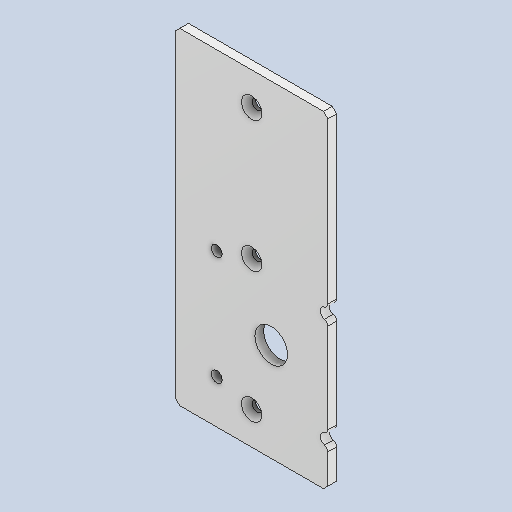
# Autodesk Inventor part: Espaçador módulo AC
Saved by Autodesk Inventor 2026 (Build 300175050, 175E)
## iProperties
Created: 2025-08-25
Part Number: Espaçador módulo AC
Material: Poliacetal
Document SubType Name: Modeling
Designer: Kedson Neves
Density: 1.41 g/cm^3
Appearance: Suave - Branco
Description: Espaçador módulo AC
Author: Kedson Neves
Autodesk Inventor part; units mm, degrees
ref_plane "YZ Plane" through (0, 0, 0) normal (1, 0, 0) x (0, 1, 0)
ref_plane "XZ Plane" through (0, 0, 0) normal (0, 1, 0) x (-1, 0, 0)
ref_plane "XY Plane" through (0, 0, 0) normal (0, 0, 1) x (1, 0, 0)
sketch "Esboço1" plane through (0, 0, 0) normal (0, 0, 1) x (1, 0, 0)
  line L0 (-35, -75) -> (35, -75)
  line L1 (35, -75) -> (35, 75)
  line L2 (35, 75) -> (-35, 75)
  line L3 (-35, 75) -> (-35, -75)
  line L4 (-35, -75) -> (35, 75) construction
  line L5 (35, -75) -> (-35, 75) construction
  point P0 (0, 0)
  dimension "d0" = 150
  dimension "d1" = 70
  constraints: 12 end point, 2 midpoint, 2 parallel, 1 horizontal, 1 perpendicular
  measures "d0" distance of L2.end L0.start
  measures "d1" distance of L1.end L2.end
extrude "Extrusão1" add sketch "Esboço1" along normal blind 4
sketch "Esboço2" plane through (0, 0, 4) normal (0, 0, 1) x (1, 0, 0)
  line L0 (35, 75) -> (-35, 75) projected
  line L1 (-35, -75) -> (35, -75) projected
  line L2 (-35, 75) -> (-35, -75) projected
  point P0 (0, 0)
  point P1 (0, 60)
  point P2 (0, -60)
  point P3 (0, 0)
  dimension "d4" = 15
  dimension "d5" = 15
  dimension "d6" = 35
  dimension "d7" = 35
  constraints: 1 coincident
  measures "d4" distance from line of L0 point (0, 60)
  measures "d5" distance from line of L1 point (0, -60)
  measures "d6" distance from line of L2 point (0, -60)
  measures "d7" distance from line of L2 point (0, 60)
hole "Furo1" at (0, 60, 4) at (0, -60, 4) at (0, 0, 4) direction (0, 0, -1) diameter 4.5 end through all countersink diameter 9.4 countersink angle 90 clearance for "Countersunk Flat Head Screw ISO 2009/7046" size "M4" standard "ISO"
chamfer "Chanfro1" distance 2 angle 45 4 edges at (35, -75, 2) (-35, -75, 2) (35, 75, 2) (-35, 75, 2)
sketch "Esboço3" plane through (0, 0, 4) normal (0, 0, 1) x (1, 0, 0)
  circle A0 centre (34, -55) radius 1.5706 projected
  circle A1 centre (34, -5) radius 1.5706 projected
  circle A2 centre (-16, -55) radius 3.8 construction
  circle A3 centre (-16, -55) radius 2.2 construction
  circle A4 centre (-16, -5) radius 3.8 construction
  circle A5 centre (34, -55) radius 2.5
  circle A6 centre (34, -5) radius 2.5
  circle A7 centre (-16, -55) radius 2.5
  circle A8 centre (-16, -5) radius 2.5
  point P0 (0, 0)
  dimension "d18" = 5
  constraints: 4 centre point, 4 coincident, 3 equal radius
  measures "d18" diameter of A5
extrude "Extrusão2" cut sketch "Esboço3" against normal blind 10 contours A0 | A1 | A5 | A6 | A7 | A8
fillet "Arredondamento1" radius 2 4 edges at (35, -2.7087, 2) (35, -7.2913, 2) (35, -52.7087, 2) (35, -57.2913, 2)
sketch "Esboço4" plane through (0, 0, 4) normal (0, 0, 1) x (1, 0, 0)
  circle A0 centre (9, -30) radius 5.5 projected
  circle A1 centre (9, -30) radius 7.5
  point P0 (0, 0)
  dimension "d22" = 15
  constraints: 1 centre point, 1 coincident
  measures "d22" diameter of A1
extrude "Extrusão3" cut sketch "Esboço4" against normal through all contours A0 | A1
